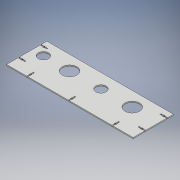
# Autodesk Inventor part: P1
Saved by Autodesk Inventor 2018 (Build 220112000, 112)
## iProperties
Created: 2018-02-28
Part Number: P1
Material: Generic
Document SubType Name: Modeling
Designer: isai
Density: 1 g/cm^3
Appearance: Default
Author: isai
Autodesk Inventor part; units mm, degrees
ref_plane "YZ Plane" through (0, 0, 0) normal (1, 0, 0) x (0, 1, 0)
ref_plane "XZ Plane" through (0, 0, 0) normal (0, 1, 0) x (-1, 0, 0)
ref_plane "XY Plane" through (0, 0, 0) normal (0, 0, 1) x (1, 0, 0)
sketch "Sketch2" plane through (0, 0, 0) normal (0, 0, 1) x (1, 0, 0)
  line L0 (220, -70) -> (-220, -70)
  line L1 (-220, -70) -> (-220, 70)
  line L2 (-220, 70) -> (220, 70)
  line L3 (220, 70) -> (220, -70)
  line L4 (220, -70) -> (-220, 70) construction
  line L5 (-220, -70) -> (220, 70) construction
  point P0 (0, 0)
  dimension "d8" = 440
  dimension "d9" = 140
  constraints: 12 end point, 2 midpoint, 2 parallel, 1 horizontal, 1 perpendicular
  measures "d8" distance of L1.end L2.end
  measures "d9" distance of L0.end L1.end
extrude "Extrusion2" add sketch "Sketch2" along normal blind 4
sketch "Sketch3" plane through (0, 0, 4) normal (0, 0, 1) x (1, 0, 0)
  line L0 (-220, -70) -> (220, -70) projected
  line L1 (220, -70) -> (220, 70) projected
  line L2 (220, 70) -> (-220, 70) projected
  line L3 (-220, 70) -> (-220, -70) projected
  circle A0 centre (-182, 20) radius 18
  circle A1 centre (-91, 20) radius 25.5
  circle A2 centre (18, 20) radius 18
  circle A3 centre (127, 20) radius 25.5
  point P0 (0, 0)
  dimension "d13" = 91
  dimension "d14" = 36
  dimension "d15" = 51
  dimension "d16" = 38
  dimension "d17" = 109
  dimension "d18" = 36
  dimension "d19" = 109
  dimension "d20" = 51
  dimension "d23" = 50
  constraints: 4 centre point, 2 coincident
  measures "d13" distance of A1.centre A0.centre
  measures "d14" diameter of A0
  measures "d15" diameter of A1
  measures "d16" distance from line of A0.centre L3
  measures "d17" distance of point (18, 20) A1.centre
  measures "d18" diameter of A2
  measures "d19" distance of point (127, 20) point (18, 20)
  measures "d20" diameter of A3
  measures "d23" distance from line of L2 A0.centre
extrude "Extrusion3" cut sketch "Sketch3" against normal blind 4 contours A0 | A1 | A2 | A3
sketch "Sketch4" plane through (0, 0, 4) normal (0, 0, 1) x (1, 0, 0)
  circle A0 centre (127, 20) radius 25.5
  circle A1 centre (18, 20) radius 25.5
  circle A2 centre (-91, 20) radius 18
  circle A3 centre (-182, 20) radius 18
  line L0 (-220, 70) -> (220, 70)
  line L1 (220, 70) -> (220, -70)
  line L2 (220, -70) -> (-220, -70)
  line L3 (-220, -70) -> (-220, 70)
  line L4 (220, 70) -> (224, 70)
  line L5 (224, -62.3) -> (220, -62.3)
  line L6 (224, 50) -> (197, 50)
  line L7 (197, 50) -> (197, 46.4)
  line L8 (197, 46.4) -> (224, 46.4)
  line L9 (224, 46.4) -> (224, 50)
  line L10 (210, 45.2) -> (207, 45.2)
  line L11 (207, 45.2) -> (207, 51.2)
  line L12 (207, 51.2) -> (210, 51.2)
  line L13 (210, 51.2) -> (210, 45.2)
  line L14 (210, 45.2) -> (207, 51.2) construction
  line L15 (207, 45.2) -> (210, 51.2) construction
  line L16 (224, -26.4) -> (197, -26.4)
  line L17 (197, -26.4) -> (197, -30)
  line L18 (197, -30) -> (224, -30)
  line L19 (224, -30) -> (224, -26.4)
  line L20 (210, -31.2) -> (207, -31.2)
  line L21 (207, -31.2) -> (207, -25.2)
  line L22 (207, -25.2) -> (210, -25.2)
  line L23 (210, -25.2) -> (210, -31.2)
  line L24 (210, -31.2) -> (207, -25.2) construction
  line L25 (207, -31.2) -> (210, -25.2) construction
  line L26 (224, 70) -> (224, 46.4)
  line L27 (224, -26.4) -> (224, -30)
  line L28 (220, -62.3) -> (220, -30)
  point P0 (0, 0)
  point P1 (208.5, 48.2)
  point P2 (208.5, -28.2)
  point P3 (220, 46.4)
  point P4 (220, -26.4)
  dimension "d24" = 4
  dimension "d25" = 27
  dimension "d26" = 3.6
  dimension "d27" = 3
  dimension "d28" = 6
  dimension "d29" = 10
  dimension "d30" = 140
  dimension "d31" = 20
  dimension "d32" = 27
  dimension "d33" = 3
  dimension "d34" = 6
  dimension "d35" = 40
  dimension "d36" = 3.6
  constraints: 58 end point, 11 parallel, 6 perpendicular, 5 horizontal, 4 centre point, 4 midpoint, 4 point on line
  measures "d24" distance of L5.start L28.start
  measures "d25" distance of L8.end L7.end
  measures "d26" distance of L7.end L6.end
  measures "d27" distance of L11.end L12.end
  measures "d28" distance of L10.end L11.end
  measures "d29" distance between parallel lines of L1 L13
  measures "d30" distance between parallel lines of L2 L0
  measures "d31" distance between parallel lines of L6 L0
  measures "d32" distance of L18.end L17.end
  measures "d33" distance of L22.start L22.end
  measures "d34" distance of L21.start L22.start
  measures "d35" distance between parallel lines of L2 L18
  measures "d36" distance of L17.start L17.end
extrude "Extrusion4" cut sketch "Sketch4" against normal blind 4 contours L6 L9 L8 L1 | L1 L8 L13 L6 | L13 L8 L11 L6 | L6 L11 L12 L13 | L16 L19 L18 L1 | L1 L18 L23 L16 | L13 L10 L11 L8 | L11 L8 L7 L6 | L23 L18 L21 L16 | L16 L21 L22 L23 | L23 L20 L21 L18 | L21 L18 L17 L16
ref_plane "Work Plane1" through (0, 70, 4) normal (1, 0, 0) x (0, 0, -1)
mirror "Mirror1" about plane through (0, 70, 4) normal (1, 0, 0) of "Extrusion4"
sketch "Sketch5" plane through (0, 0, 4) normal (0, 0, 1) x (1, 0, 0)
  line L0 (-224, -46) -> (-220, -46)
  line L1 (-224, -50) -> (-224, -46)
  line L2 (-220, -50) -> (-224, -50)
  line L3 (-220, -50) -> (-220, -70)
  line L4 (-220, -70) -> (220, -70)
  line L5 (220, -70) -> (220, -50)
  line L6 (220, -50) -> (224, -50)
  line L7 (224, -50) -> (224, -46)
  line L8 (224, -46) -> (220, -46)
  line L9 (-150, -57) -> (-150, -47)
  line L10 (-151.2, -57) -> (-150, -57)
  line L11 (-150, -47) -> (-146.4, -47)
  line L12 (-146.4, -47) -> (-146.4, -57)
  line L13 (-146.4, -57) -> (-145.2, -57)
  line L14 (-150, -60) -> (-151.2, -60)
  line L15 (-151.2, -60) -> (-151.2, -57)
  line L16 (-145.2, -57) -> (-145.2, -60)
  line L17 (-145.2, -60) -> (-146.4, -60)
  line L18 (-150, -70) -> (-150, -60)
  line L19 (-146.4, -60) -> (-146.4, -70)
  line L20 (-146.4, -70) -> (-150, -70)
  line L21 (-220, -70) -> (220, -70)
  line L22 (151.2, -57) -> (151.2, -60)
  line L23 (150, -57) -> (151.2, -57)
  line L24 (150, -47) -> (150, -57)
  line L25 (146.4, -47) -> (150, -47)
  line L26 (150, -60) -> (150, -70)
  line L27 (146.4, -57) -> (146.4, -47)
  line L28 (146.4, -70) -> (146.4, -60)
  line L29 (145.2, -57) -> (146.4, -57)
  line L30 (145.2, -60) -> (145.2, -57)
  line L31 (146.4, -60) -> (145.2, -60)
  line L32 (151.2, -60) -> (150, -60)
  line L33 (150, -70) -> (146.4, -70)
  line L34 (-0.6, -57) -> (-0.6, -60)
  line L35 (-1.8, -57) -> (-0.6, -57)
  line L36 (-1.8, -47) -> (-1.8, -57)
  line L37 (-5.4, -47) -> (-1.8, -47)
  line L38 (-1.8, -60) -> (-1.8, -70)
  line L39 (-5.4, -57) -> (-5.4, -47)
  line L40 (-5.4, -70) -> (-5.4, -60)
  line L41 (-6.6, -57) -> (-5.4, -57)
  line L42 (-6.6, -60) -> (-6.6, -57)
  line L43 (-5.4, -60) -> (-6.6, -60)
  line L44 (-0.6, -60) -> (-1.8, -60)
  line L45 (-1.8, -70) -> (-5.4, -70)
  line L46 (-220, -70) -> (220, -70) projected
  point P0 (0, 0)
  point P1 (-143.2198, -70)
  point P2 (176.1378, -65.3908)
  point P3 (10.9651, -65.3908)
  dimension "d39" = 70
  dimension "d40" = 3.6
  dimension "d41" = 3.6
  dimension "d42" = 6
  dimension "d43" = 1.2
  dimension "d44" = 3
  dimension "d45" = 1.2
  dimension "d46" = 3.6
  dimension "d47" = 3.6
  dimension "d48" = 6
  dimension "d49" = 1.2
  dimension "d50" = 3
  dimension "d51" = 1.2
  dimension "d52" = 3.6
  dimension "d53" = 3.6
  dimension "d54" = 6
  dimension "d55" = 1.2
  dimension "d56" = 3
  dimension "d57" = 1.2
  dimension "d58" = 70
  dimension "d59" = 440
  dimension "d60" = 221.8
  constraints: 92 end point, 18 perpendicular, 3 parallel, 1 point on line
  measures "d39" distance between parallel lines of L18 L3
  measures "d40" distance between parallel lines of L19 L18
  measures "d41" distance between parallel lines of L12 L9
  measures "d42" distance between parallel lines of L16 L15
  measures "d43" distance between parallel lines of L15 L9
  measures "d44" distance between parallel lines of L14 L10
  measures "d45" distance between parallel lines of L18 L15
  measures "d46" distance between parallel lines of L26 L28
  measures "d47" distance between parallel lines of L24 L27
  measures "d48" distance between parallel lines of L22 L30
  measures "d49" distance between parallel lines of L30 L27
  measures "d50" distance between parallel lines of L31 L29
  measures "d51" distance between parallel lines of L28 L30
  measures "d52" distance between parallel lines of L38 L40
  measures "d53" distance between parallel lines of L36 L39
  measures "d54" distance between parallel lines of L34 L42
  measures "d55" distance between parallel lines of L42 L39
  measures "d56" distance between parallel lines of L43 L41
  measures "d57" distance between parallel lines of L40 L42
  measures "d58" distance between parallel lines of L5 L26
  measures "d59" distance between parallel lines of L5 L3
  measures "d60" distance between parallel lines of L5 L38
extrude "Extrusion5" cut sketch "Sketch5" against normal blind 10
body "Solid2"
